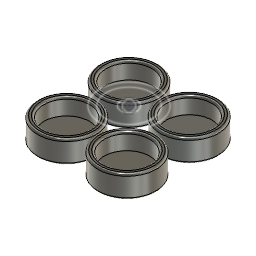
isaac-damian-wheel (Autodesk Fusion 360 design; units mm, degrees)
Autodesk Fusion 360 part; units mm, degrees
sketch "Sketch1" plane through (0, 0, 0) normal (0, 0, 1) x (1, 0, 0)
  circle A0 centre (0, 0) radius 11
  circle A1 centre (0, 0) radius 4
  circle A2 centre (0, 0) radius 14
  dimension "d1" = 22
  dimension "d2" = 8
  dimension "d3" = 3
  constraint coincident A0.centre A1.centre
  measures "d1" diameter of A0
  measures "d2" diameter of A1
extrude "Extrude1" add sketch "Sketch1" along normal blind 3 contours A0 makes body 1
extrude "Extrude2" add sketch "Sketch1" along normal blind 11 contours A2 bodies 1
delete_face "DeleteFace1" 1 faces at (3.995, -0.1994, 2) on bodies 1
copy_body "CopyPasteBodies1" bodies 1 makes body 2
move_body "Move1" bodies 2 to x (1, 0, 0) y (0, 1, 0) z (0, 0, 1) at (29, 0, 0)
copy_body "CopyPasteBodies2" bodies 2 1 makes body 3 makes body 4
move_body "Move2" bodies 3 4 to x (1, 0, 0) y (0, 1, 0) z (0, 0, 1) at (0, -30, 0)
sketch "Sketch2" plane through (0, 0, 0) normal (0, 0, -1) x (1, 0, 0)
  circle A0 centre (29, 0) radius 14
fillet "Fillet1" radius 1 12 edges at (-10.2556, 3.9778, 11) (-13.0526, -5.0626, 11) (-13.0526, -5.0626, 0) (18.7444, 3.9778, 11) (15.9474, -5.0626, 11) (15.9474, -5.0626, 0) (15.9474, -35.0626, 11) (18.7444, -26.0222, 11) (15.9474, -35.0626, 0) (-10.2556, -26.0222, 11) (-13.0526, -35.0626, 11) (-13.0526, -35.0626, 0) on bodies 1 2 3 4
